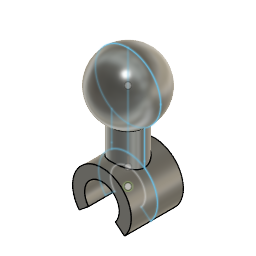
Coupler (Autodesk Fusion 360 design; units mm, degrees)
Autodesk Fusion 360 part; units mm, degrees
note: some values were not read from the file. Set by a fixed rule: which sketch regions a step uses.
sketch "Sketch1" plane through (0, 0, 0) normal (0, 1, 0) x (1, 0, 0)
  arc A0 (-1.25, -15.8708) -> (1.25, -15.8708) centre (0, -14) ccw
  line L0 (0, -16.25) -> (0, -18.2)
  line L1 (0, -15.3) -> (0, -16.25) construction
  line L2 (-1.25, -15.8708) -> (-1.25, -16.3)
  line L3 (-1.25, -16.3) -> (-1.25, -18.5349)
  line L4 (1.25, -15.8708) -> (1.25, -16.3)
  line L5 (1.25, -16.3) -> (1.25, -18.5349)
  circle A1 centre (0, -20.7) radius 2.5
  line L6 (0, -18.2) -> (0, -23.2)
  line L7 (-1.0225, -13.1573) -> (-1.7363, -12.569)
  line L8 (1.0225, -13.1573) -> (1.7363, -12.569)
  arc A2 (-1.0225, -13.1573) -> (1.0225, -13.1573) centre (0, -14) ccw
  arc A3 (-1.7363, -12.569) -> (1.7363, -12.569) centre (0, -14) ccw
  dimension "d5" = 5
  dimension "d9" = 2.65
  constraint vertical L0
  constraint coincident A1 L3.end
  constraint coincident A1 L0.end
  constraint coincident A1 L5.end
  constraint coincident A1 L6.end
  constraint parallel L0 L6
  constraint coincident A0 L0.start
  constraint concentric A0 A2
  constraint coincident A0.start A3
  constraint concentric A2 A3
  measures "d5" diameter of A1
  measures "d9" diameter of A2
revolve "Revolve1" add sketch "Sketch1" angle 360 about axis through (0, 0, 18.2) along (0, 0, 1) contours A0 L0 L4 L5 A1 A3 | A1 L6 picked at (0.9452, -20.1531)
extrude "Extrude1" add sketch "Sketch1" along normal mid plane 4 contours A0 L7 L8 A2 A3
